Autodesk Inventor part; units mm, degrees
(part 3 of 5)
  line L1792 (36.1896, -14.5898) -> (36.2262, -14.8073)
  line L1793 (36.1751, -14.3579) -> (36.1896, -14.5898)
  line L1794 (36.1824, -14.1175) -> (36.1751, -14.3579)
  line L1795 (36.2227, -13.8474) -> (36.1824, -14.1175)
  line L1796 (36.3174, -13.5133) -> (36.2227, -13.8474)
  line L1797 (36.3367, -13.4614) -> (36.3174, -13.5133)
  line L1798 (36.3559, -13.4094) -> (36.3367, -13.4614)
  line L1799 (36.375, -13.3574) -> (36.3559, -13.4094)
  line L1800 (36.3941, -13.3053) -> (36.375, -13.3574)
  line L1801 (36.4131, -13.2533) -> (36.3941, -13.3053)
  circle A36 centre (0, 0) radius 4
  dimension "d26" = 8
  constraints: 3604 end point, 50 symmetric about line, 37 centre point, 4 midpoint, 1 coincident, 1 point on line, 1 other
  measures "d26" diameter of A36
extrude "押し出し1" add sketch "スケッチ1" along normal blind 3
sketch "スケッチ3" plane through (0, 0, 0) normal (0, 0, -1) x (-1, 0, 0)
  circle A0 centre (-26.7924, 20.9325) radius 1.6 projected
  circle A1 centre (-38.6125, 30.1674) radius 1.6 projected
  line L0 (-15.8708, 21.9173) -> (-25.1057, 10.0971) projected
  line L1 (-15.8708, 21.9173) -> (-140.3765, 119.1918) projected
  line L2 (-149.6114, 107.3716) -> (-140.3765, 119.1918) projected
  line L3 (-25.1057, 10.0971) -> (-149.6114, 107.3716) projected
  circle A2 centre (-9.3717, 32.6829) radius 1.6 projected
  circle A3 centre (-13.5062, 47.1018) radius 1.6 projected
  line L4 (0.0429, 27.0601) -> (-14.376, 22.9255) projected
  line L5 (0.0429, 27.0601) -> (-55.0846, 219.3124) projected
  line L6 (-69.5035, 215.1779) -> (-55.0846, 219.3124) projected
  line L7 (-14.376, 22.9255) -> (-69.5035, 215.1779) projected
  arc A4 (-9.1991, 59.2906) -> (-51.5273, 30.7399) centre (0, 0) ccw
  line L8 (-51.5273, 30.7399) -> (-25.1057, 10.0971)
  line L9 (-9.1991, 59.2906) -> (0.0429, 27.0601)
  line L10 (-25.1057, 10.0971) -> (0.0429, 27.0601)
  dimension "d23" = 60
  constraints: 6 end point, 2 point on circle, 2 point on line, 1 centre point, 1 coincident, 1 collinear, 1 perpendicular
  measures "d23" radius of A4
extrude "押し出し2" add sketch "スケッチ3" against normal blind 3 contours A0 | A1 | L1 A4 L7 L4 L10 L0 | L0 L3 A4 L1 | L4 L7 A4 L5 | A2 | A3
sketch "スケッチ2" plane through (0, 0, 0) normal (0, 0, -1) x (-1, 0, 0)
  line L0 (-25.1057, 10.0971) -> (-15.8708, 21.9173)
  line L1 (-15.8708, 21.9173) -> (-140.3765, 119.1918)
  line L2 (-140.3765, 119.1918) -> (-149.6114, 107.3716)
  line L3 (-149.6114, 107.3716) -> (-25.1057, 10.0971)
  line L4 (-20.4883, 16.0072) -> (0, 0)
  line L5 (0, 0) -> (0, 26)
  line L6 (0, 0) -> (-9.3717, 32.6829)
  point P0 (-26.7924, 20.9325)
  point P1 (-38.6125, 30.1674)
  point P2 (-13.5062, 47.1018)
  dimension "d6" = 158
  dimension "d7" = 15
  dimension "d8" = 52
  dimension "d9" = 26
  dimension "d10" = 15
  dimension "d11" = 8
  dimension "d42" = 15
  dimension "d43" = 34
  dimension "d44" = 36
  constraints: 14 end point, 3 point on line, 2 parallel, 2 perpendicular, 1 equal length, 1 midpoint, 1 vertical
  measures "d6" distance of L1.end L0.end
  measures "d7" distance of L1.end L2.end
  measures "d8" angle of L4 L5
  measures "d9" distance of L4.start L4.end
  measures "d10" distance of point (-38.613, 30.167) point (-26.792, 20.932)
  measures "d11" distance from line of point (-26.792, 20.932) L0
  measures "d42" distance of point (-13.506, 47.102) L6.end
  measures "d43" distance of L4.end L6.end
  measures "d44" angle of L4 L6
hole "穴1" at (26.7924, 20.9325, 0) at (38.6125, 30.1674, 0) at (9.3717, 32.6829, 0) at (13.5062, 47.1018, 0) direction (0, 0, 1) diameter 2.459 end through all thread size "M3x0.5" class "6H" standard "ISO Metric profile"
sketch "スケッチ4" plane through (0, 0, 0) normal (0, 0, -1) x (-1, 0, 0)
  circle A0 centre (-9.3717, 32.6829) radius 1.2295 projected
  circle A1 centre (-26.7924, 20.9325) radius 1.2295 projected
  circle A2 centre (-38.6125, 30.1674) radius 1.2295 projected
  circle A3 centre (-13.5062, 47.1018) radius 1.2295 projected
  line L0 (-43.4971, 24.2746) -> (-43.4223, 24.4075) projected
  line L1 (-43.6728, 23.957) -> (-43.4971, 24.2746) projected
  line L2 (-43.8463, 23.638) -> (-43.6728, 23.957) projected
  line L3 (-44.0174, 23.3178) -> (-43.8463, 23.638) projected
  line L4 (-43.7924, 22.9383) -> (-44.0174, 23.3178) projected
  line L5 (-43.5626, 22.5656) -> (-43.7924, 22.9383) projected
  line L6 (-43.3282, 22.1998) -> (-43.5626, 22.5656) projected
  line L7 (-43.0891, 21.841) -> (-43.3282, 22.1998) projected
  line L8 (-42.8453, 21.4895) -> (-43.0891, 21.841) projected
  line L9 (-42.5969, 21.1453) -> (-42.8453, 21.4895) projected
  line L10 (-42.3439, 20.8086) -> (-42.5969, 21.1453) projected
  line L11 (-42.0862, 20.4798) -> (-42.3439, 20.8086) projected
  line L12 (-41.8239, 20.1589) -> (-42.0862, 20.4798) projected
  line L13 (-41.5569, 19.8464) -> (-41.8239, 20.1589) projected
  line L14 (-41.2851, 19.5423) -> (-41.5569, 19.8464) projected
  line L15 (-41.0086, 19.2472) -> (-41.2851, 19.5423) projected
  line L16 (-40.7272, 18.9615) -> (-41.0086, 19.2472) projected
  line L17 (-40.4408, 18.6855) -> (-40.7272, 18.9615) projected
  line L18 (-40.1491, 18.4201) -> (-40.4408, 18.6855) projected
  line L19 (-39.852, 18.1659) -> (-40.1491, 18.4201) projected
  line L20 (-39.5489, 17.9241) -> (-39.852, 18.1659) projected
  line L21 (-39.2392, 17.6965) -> (-39.5489, 17.9241) projected
  line L22 (-38.9217, 17.4859) -> (-39.2392, 17.6965) projected
  line L23 (-38.5928, 17.3007) -> (-38.9217, 17.4859) projected
  line L24 (-38.3425, 17.1764) -> (-38.5928, 17.3007) projected
  line L25 (-38.105, 17.0451) -> (-38.3425, 17.1764) projected
  line L26 (-37.8794, 16.9086) -> (-38.105, 17.0451) projected
  line L27 (-37.6648, 16.7698) -> (-37.8794, 16.9086) projected
  line L28 (-37.4636, 16.6236) -> (-37.6648, 16.7698) projected
  line L29 (-37.2761, 16.4698) -> (-37.4636, 16.6236) projected
  line L30 (-37.1025, 16.3084) -> (-37.2761, 16.4698) projected
  line L31 (-36.9406, 16.1452) -> (-37.1025, 16.3084) projected
  line L32 (-36.7931, 15.9746) -> (-36.9406, 16.1452) projected
  line L33 (-36.6611, 15.7947) -> (-36.7931, 15.9746) projected
  line L34 (-36.5421, 15.6124) -> (-36.6611, 15.7947) projected
  line L35 (-36.4388, 15.4218) -> (-36.5421, 15.6124) projected
  line L36 (-36.3516, 15.2235) -> (-36.4388, 15.4218) projected
  line L37 (-36.2795, 15.0209) -> (-36.3516, 15.2235) projected
  line L38 (-36.2262, 14.8073) -> (-36.2795, 15.0209) projected
  line L39 (-36.1896, 14.5898) -> (-36.2262, 14.8073) projected
  line L40 (-36.1751, 14.3579) -> (-36.1896, 14.5898) projected
  line L41 (-36.1824, 14.1175) -> (-36.1751, 14.3579) projected
  line L42 (-36.2227, 13.8474) -> (-36.1824, 14.1175) projected
  line L43 (-36.3174, 13.5133) -> (-36.2227, 13.8474) projected
  line L44 (-36.3367, 13.4614) -> (-36.3174, 13.5133) projected
  line L45 (-36.3559, 13.4094) -> (-36.3367, 13.4614) projected
  line L46 (-36.375, 13.3574) -> (-36.3559, 13.4094) projected
  line L47 (-36.3941, 13.3053) -> (-36.375, 13.3574) projected
  line L48 (-36.4131, 13.2533) -> (-36.3941, 13.3053) projected
  line L49 (-36.432, 13.2012) -> (-36.4131, 13.2533) projected
  line L50 (-36.4508, 13.1491) -> (-36.432, 13.2012) projected
  line L51 (-36.4696, 13.0969) -> (-36.4508, 13.1491) projected
  line L52 (-36.4883, 13.0448) -> (-36.4696, 13.0969) projected
  line L53 (-36.5069, 12.9926) -> (-36.4883, 13.0448) projected
  line L54 (-36.6492, 12.6758) -> (-36.5069, 12.9926) projected
  line L55 (-36.7919, 12.4429) -> (-36.6492, 12.6758) projected
  line L56 (-36.9408, 12.2541) -> (-36.7919, 12.4429) projected
  line L57 (-37.1009, 12.0858) -> (-36.9408, 12.2541) projected
  line L58 (-37.2688, 11.9427) -> (-37.1009, 12.0858) projected
  line L59 (-37.447, 11.8133) -> (-37.2688, 11.9427) projected
  line L60 (-37.6324, 11.7044) -> (-37.447, 11.8133) projected
  line L61 (-37.8267, 11.6087) -> (-37.6324, 11.7044) projected
  line L62 (-38.0283, 11.529) -> (-37.8267, 11.6087) projected
  line L63 (-38.2367, 11.4659) -> (-38.0283, 11.529) projected
  line L64 (-38.4534, 11.4129) -> (-38.2367, 11.4659) projected
  line L65 (-38.6761, 11.377) -> (-38.4534, 11.4129) projected
  line L66 (-38.905, 11.3561) -> (-38.6761, 11.377) projected
  line L67 (-39.1417, 11.344) -> (-38.905, 11.3561) projected
  line L68 (-39.3842, 11.3467) -> (-39.1417, 11.344) projected
  line L69 (-39.6323, 11.364) -> (-39.3842, 11.3467) projected
  line L70 (-39.886, 11.3956) -> (-39.6323, 11.364) projected
  line L71 (-40.1465, 11.4361) -> (-39.886, 11.3956) projected
  line L72 (-40.4129, 11.4882) -> (-40.1465, 11.4361) projected
  line L73 (-40.6845, 11.5538) -> (-40.4129, 11.4882) projected
  line L74 (-41.0555, 11.6234) -> (-40.6845, 11.5538) projected
  line L75 (-41.4341, 11.6662) -> (-41.0555, 11.6234) projected
  line L76 (-41.8176, 11.6908) -> (-41.4341, 11.6662) projected
  line L77 (-42.2052, 11.7005) -> (-41.8176, 11.6908) projected
  line L78 (-42.5962, 11.6968) -> (-42.2052, 11.7005) projected
  line L79 (-42.9903, 11.6809) -> (-42.5962, 11.6968) projected
  line L80 (-43.387, 11.6536) -> (-42.9903, 11.6809) projected
  line L81 (-43.7863, 11.6156) -> (-43.387, 11.6536) projected
  line L82 (-44.1878, 11.5673) -> (-43.7863, 11.6156) projected
  line L83 (-44.5914, 11.509) -> (-44.1878, 11.5673) projected
  line L84 (-44.9969, 11.4412) -> (-44.5914, 11.509) projected
  line L85 (-45.4041, 11.3641) -> (-44.9969, 11.4412) projected
  line L86 (-45.8128, 11.2778) -> (-45.4041, 11.3641) projected
  line L87 (-46.223, 11.1825) -> (-45.8128, 11.2778) projected
  line L88 (-46.6346, 11.0786) -> (-46.223, 11.1825) projected
  line L89 (-47.0473, 10.9659) -> (-46.6346, 11.0786) projected
  line L90 (-47.4611, 10.8448) -> (-47.0473, 10.9659) projected
  line L91 (-47.8758, 10.7152) -> (-47.4611, 10.8448) projected
  line L92 (-48.2914, 10.5774) -> (-47.8758, 10.7152) projected
  line L93 (-48.7077, 10.4313) -> (-48.2914, 10.5774) projected
  line L94 (-48.7824, 10.0761) -> (-48.7077, 10.4313) projected
  line L95 (-48.8546, 9.7203) -> (-48.7824, 10.0761) projected
  line L96 (-48.9241, 9.3639) -> (-48.8546, 9.7203) projected
  line L97 (-48.9911, 9.0071) -> (-48.9241, 9.3639) projected
  line L98 (-49.0554, 8.6498) -> (-48.9911, 9.0071) projected
  line L99 (-49.1172, 8.292) -> (-49.0554, 8.6498) projected
  line L100 (-49.1763, 7.9338) -> (-49.1172, 8.292) projected
  line L101 (-49.2328, 7.5752) -> (-49.1763, 7.9338) projected
  line L102 (-49.2867, 7.2162) -> (-49.2328, 7.5752) projected
  line L103 (-49.338, 6.8568) -> (-49.2867, 7.2162) projected
  line L104 (-48.9968, 6.5771) -> (-49.338, 6.8568) projected
  line L105 (-48.6534, 6.3055) -> (-48.9968, 6.5771) projected
  line L106 (-48.308, 6.0419) -> (-48.6534, 6.3055) projected
  line L107 (-47.9606, 5.7865) -> (-48.308, 6.0419) projected
  line L108 (-47.6113, 5.5395) -> (-47.9606, 5.7865) projected
  line L109 (-47.2601, 5.3011) -> (-47.6113, 5.5395) projected
  line L110 (-46.9072, 5.0713) -> (-47.2601, 5.3011) projected
  line L111 (-46.5526, 4.8504) -> (-46.9072, 5.0713) projected
  line L112 (-46.1963, 4.6386) -> (-46.5526, 4.8504) projected
  line L113 (-45.8385, 4.4362) -> (-46.1963, 4.6386) projected
  line L114 (-45.4792, 4.2434) -> (-45.8385, 4.4362) projected
  line L115 (-45.1184, 4.0607) -> (-45.4792, 4.2434) projected
  line L116 (-44.7563, 3.8884) -> (-45.1184, 4.0607) projected
  line L117 (-44.3927, 3.7271) -> (-44.7563, 3.8884) projected
  line L118 (-44.0279, 3.5774) -> (-44.3927, 3.7271) projected
  line L119 (-43.6617, 3.4402) -> (-44.0279, 3.5774) projected
  line L120 (-43.2942, 3.3167) -> (-43.6617, 3.4402) projected
  line L121 (-42.9254, 3.2087) -> (-43.2942, 3.3167) projected
  line L122 (-42.555, 3.1194) -> (-42.9254, 3.2087) projected
  line L123 (-42.1825, 3.0578) -> (-42.555, 3.1194) projected
  line L124 (-41.9049, 3.0266) -> (-42.1825, 3.0578) projected
  line L125 (-41.6367, 2.9845) -> (-41.9049, 3.0266) projected
  line L126 (-41.3781, 2.9334) -> (-41.6367, 2.9845) projected
  line L127 (-41.1289, 2.8764) -> (-41.3781, 2.9334) projected
  line L128 (-40.8898, 2.8078) -> (-41.1289, 2.8764) projected
  line L129 (-40.661, 2.7274) -> (-40.8898, 2.8078) projected
  line L130 (-40.4428, 2.6351) -> (-40.661, 2.7274) projected
  line L131 (-40.2348, 2.5371) -> (-40.4428, 2.6351) projected
  line L132 (-40.0379, 2.4272) -> (-40.2348, 2.5371) projected
  line L133 (-39.8523, 2.3033) -> (-40.0379, 2.4272) projected
  line L134 (-39.6781, 2.1727) -> (-39.8523, 2.3033) projected
  line L135 (-39.5158, 2.0289) -> (-39.6781, 2.1727) projected
  line L136 (-39.366, 1.8725) -> (-39.5158, 2.0289) projected
  line L137 (-39.2291, 1.7067) -> (-39.366, 1.8725) projected
  line L138 (-39.1059, 1.5242) -> (-39.2291, 1.7067) projected
  line L139 (-38.997, 1.3323) -> (-39.1059, 1.5242) projected
  line L140 (-38.9042, 1.1194) -> (-38.997, 1.3323) projected
  line L141 (-38.8288, 0.891) -> (-38.9042, 1.1194) projected
  line L142 (-38.7743, 0.6234) -> (-38.8288, 0.891) projected
  line L143 (-38.749, 0.2771) -> (-38.7743, 0.6234) projected
  line L144 (-38.7494, 0.2217) -> (-38.749, 0.2771) projected
  line L145 (-38.7496, 0.1663) -> (-38.7494, 0.2217) projected
  line L146 (-38.7498, 0.1108) -> (-38.7496, 0.1663) projected
  line L147 (-38.75, 0.0554) -> (-38.7498, 0.1108) projected
  line L148 (-38.75, 0) -> (-38.75, 0.0554) projected
  line L149 (-38.75, -0.0554) -> (-38.75, 0) projected
  line L150 (-38.7498, -0.1108) -> (-38.75, -0.0554) projected
  line L151 (-38.7496, -0.1663) -> (-38.7498, -0.1108) projected
  line L152 (-38.7494, -0.2217) -> (-38.7496, -0.1663) projected
  line L153 (-38.749, -0.2771) -> (-38.7494, -0.2217) projected
  line L154 (-38.7743, -0.6234) -> (-38.749, -0.2771) projected
  line L155 (-38.8288, -0.891) -> (-38.7743, -0.6234) projected
  line L156 (-38.9042, -1.1194) -> (-38.8288, -0.891) projected
  line L157 (-38.997, -1.3323) -> (-38.9042, -1.1194) projected
  line L158 (-39.1059, -1.5242) -> (-38.997, -1.3323) projected
  line L159 (-39.2291, -1.7067) -> (-39.1059, -1.5242) projected
  line L160 (-39.366, -1.8725) -> (-39.2291, -1.7067) projected
  line L161 (-39.5158, -2.0289) -> (-39.366, -1.8725) projected
  line L162 (-39.6781, -2.1727) -> (-39.5158, -2.0289) projected
  line L163 (-39.8523, -2.3033) -> (-39.6781, -2.1727) projected
  line L164 (-40.0379, -2.4272) -> (-39.8523, -2.3033) projected
  line L165 (-40.2348, -2.5371) -> (-40.0379, -2.4272) projected
  line L166 (-40.4428, -2.6351) -> (-40.2348, -2.5371) projected
  line L167 (-40.661, -2.7274) -> (-40.4428, -2.6351) projected
  line L168 (-40.8898, -2.8078) -> (-40.661, -2.7274) projected
  line L169 (-41.1289, -2.8764) -> (-40.8898, -2.8078) projected
  line L170 (-41.3781, -2.9334) -> (-41.1289, -2.8764) projected
  line L171 (-41.6367, -2.9845) -> (-41.3781, -2.9334) projected
  line L172 (-41.9049, -3.0266) -> (-41.6367, -2.9845) projected
  line L173 (-42.1825, -3.0578) -> (-41.9049, -3.0266) projected
  line L174 (-42.555, -3.1194) -> (-42.1825, -3.0578) projected
  line L175 (-42.9254, -3.2087) -> (-42.555, -3.1194) projected
  line L176 (-43.2942, -3.3167) -> (-42.9254, -3.2087) projected
  line L177 (-43.6617, -3.4402) -> (-43.2942, -3.3167) projected
  line L178 (-44.0279, -3.5774) -> (-43.6617, -3.4402) projected
  line L179 (-44.3927, -3.7271) -> (-44.0279, -3.5774) projected
  line L180 (-44.7563, -3.8884) -> (-44.3927, -3.7271) projected
  line L181 (-45.1184, -4.0607) -> (-44.7563, -3.8884) projected
  line L182 (-45.4792, -4.2434) -> (-45.1184, -4.0607) projected
  line L183 (-45.8385, -4.4362) -> (-45.4792, -4.2434) projected
  line L184 (-46.1963, -4.6386) -> (-45.8385, -4.4362) projected
  line L185 (-46.5526, -4.8504) -> (-46.1963, -4.6386) projected
  line L186 (-46.9072, -5.0713) -> (-46.5526, -4.8504) projected
  line L187 (-47.2601, -5.3011) -> (-46.9072, -5.0713) projected
  line L188 (-47.6113, -5.5395) -> (-47.2601, -5.3011) projected
  line L189 (-47.9606, -5.7865) -> (-47.6113, -5.5395) projected
  line L190 (-48.308, -6.0419) -> (-47.9606, -5.7865) projected
  line L191 (-48.6534, -6.3055) -> (-48.308, -6.0419) projected
  line L192 (-48.9968, -6.5771) -> (-48.6534, -6.3055) projected
  line L193 (-49.338, -6.8568) -> (-48.9968, -6.5771) projected
  line L194 (-49.2867, -7.2162) -> (-49.338, -6.8568) projected
  line L195 (-49.2328, -7.5752) -> (-49.2867, -7.2162) projected
  line L196 (-49.1763, -7.9338) -> (-49.2328, -7.5752) projected
  line L197 (-49.1172, -8.292) -> (-49.1763, -7.9338) projected
  line L198 (-49.0554, -8.6498) -> (-49.1172, -8.292) projected
  line L199 (-48.9911, -9.0071) -> (-49.0554, -8.6498) projected
  line L200 (-48.9241, -9.3639) -> (-48.9911, -9.0071) projected
  line L201 (-48.8546, -9.7203) -> (-48.9241, -9.3639) projected
  line L202 (-48.7824, -10.0761) -> (-48.8546, -9.7203) projected
  line L203 (-48.7077, -10.4313) -> (-48.7824, -10.0761) projected
  line L204 (-48.2914, -10.5774) -> (-48.7077, -10.4313) projected
  line L205 (-47.8758, -10.7152) -> (-48.2914, -10.5774) projected
  line L206 (-47.4611, -10.8448) -> (-47.8758, -10.7152) projected
  line L207 (-47.0473, -10.9659) -> (-47.4611, -10.8448) projected
  line L208 (-46.6346, -11.0786) -> (-47.0473, -10.9659) projected
  line L209 (-46.223, -11.1825) -> (-46.6346, -11.0786) projected
  line L210 (-45.8128, -11.2778) -> (-46.223, -11.1825) projected
  line L211 (-45.4041, -11.3641) -> (-45.8128, -11.2778) projected
  line L212 (-44.9969, -11.4412) -> (-45.4041, -11.3641) projected
  line L213 (-44.5914, -11.509) -> (-44.9969, -11.4412) projected
  line L214 (-44.1878, -11.5673) -> (-44.5914, -11.509) projected
  line L215 (-43.7863, -11.6156) -> (-44.1878, -11.5673) projected
  line L216 (-43.387, -11.6536) -> (-43.7863, -11.6156) projected
  line L217 (-42.9903, -11.6809) -> (-43.387, -11.6536) projected
  line L218 (-42.5962, -11.6968) -> (-42.9903, -11.6809) projected
  line L219 (-42.2052, -11.7005) -> (-42.5962, -11.6968) projected
  line L220 (-41.8176, -11.6908) -> (-42.2052, -11.7005) projected
  line L221 (-41.4341, -11.6662) -> (-41.8176, -11.6908) projected
  line L222 (-41.0555, -11.6234) -> (-41.4341, -11.6662) projected
  line L223 (-40.6845, -11.5538) -> (-41.0555, -11.6234) projected
  line L224 (-40.4129, -11.4882) -> (-40.6845, -11.5538) projected
  line L225 (-40.1465, -11.4361) -> (-40.4129, -11.4882) projected
  line L226 (-39.886, -11.3956) -> (-40.1465, -11.4361) projected
  line L227 (-39.6323, -11.364) -> (-39.886, -11.3956) projected
  line L228 (-39.3842, -11.3467) -> (-39.6323, -11.364) projected
  line L229 (-39.1417, -11.344) -> (-39.3842, -11.3467) projected
  line L230 (-38.905, -11.3561) -> (-39.1417, -11.344) projected
  line L231 (-38.6761, -11.377) -> (-38.905, -11.3561) projected
  line L232 (-38.4534, -11.4129) -> (-38.6761, -11.377) projected
  line L233 (-38.2367, -11.4659) -> (-38.4534, -11.4129) projected
  line L234 (-38.0283, -11.529) -> (-38.2367, -11.4659) projected
  line L235 (-37.8267, -11.6087) -> (-38.0283, -11.529) projected
  line L236 (-37.6324, -11.7044) -> (-37.8267, -11.6087) projected
  line L237 (-37.447, -11.8133) -> (-37.6324, -11.7044) projected
  line L238 (-37.2688, -11.9427) -> (-37.447, -11.8133) projected
  line L239 (-37.1009, -12.0858) -> (-37.2688, -11.9427) projected
  line L240 (-36.9408, -12.2541) -> (-37.1009, -12.0858) projected
  line L241 (-36.7919, -12.4429) -> (-36.9408, -12.2541) projected
  line L242 (-36.6492, -12.6758) -> (-36.7919, -12.4429) projected
  line L243 (-36.5069, -12.9926) -> (-36.6492, -12.6758) projected
  line L244 (-36.4883, -13.0448) -> (-36.5069, -12.9926) projected
  line L245 (-36.4696, -13.0969) -> (-36.4883, -13.0448) projected
  line L246 (-36.4508, -13.1491) -> (-36.4696, -13.0969) projected
  line L247 (-36.432, -13.2012) -> (-36.4508, -13.1491) projected
  line L248 (-36.4131, -13.2533) -> (-36.432, -13.2012) projected
  line L249 (-36.3941, -13.3053) -> (-36.4131, -13.2533) projected
  line L250 (-36.375, -13.3574) -> (-36.3941, -13.3053) projected
  line L251 (-36.3559, -13.4094) -> (-36.375, -13.3574) projected
  line L252 (-36.3367, -13.4614) -> (-36.3559, -13.4094) projected
  line L253 (-36.3174, -13.5133) -> (-36.3367, -13.4614) projected
  line L254 (-36.2227, -13.8474) -> (-36.3174, -13.5133) projected
  line L255 (-36.1824, -14.1175) -> (-36.2227, -13.8474) projected
  line L256 (-36.1751, -14.3579) -> (-36.1824, -14.1175) projected
  line L257 (-36.1896, -14.5898) -> (-36.1751, -14.3579) projected
  line L258 (-36.2262, -14.8073) -> (-36.1896, -14.5898) projected
  line L259 (-36.2795, -15.0209) -> (-36.2262, -14.8073) projected
  line L260 (-36.3516, -15.2235) -> (-36.2795, -15.0209) projected
  line L261 (-36.4388, -15.4218) -> (-36.3516, -15.2235) projected
  line L262 (-36.5421, -15.6124) -> (-36.4388, -15.4218) projected
  line L263 (-36.6611, -15.7947) -> (-36.5421, -15.6124) projected
  line L264 (-36.7931, -15.9746) -> (-36.6611, -15.7947) projected
  line L265 (-36.9406, -16.1452) -> (-36.7931, -15.9746) projected
  line L266 (-37.1025, -16.3084) -> (-36.9406, -16.1452) projected
  line L267 (-37.2761, -16.4698) -> (-37.1025, -16.3084) projected
  line L268 (-37.4636, -16.6236) -> (-37.2761, -16.4698) projected
  line L269 (-37.6648, -16.7698) -> (-37.4636, -16.6236) projected
  line L270 (-37.8794, -16.9086) -> (-37.6648, -16.7698) projected
  line L271 (-38.105, -17.0451) -> (-37.8794, -16.9086) projected
  line L272 (-38.3425, -17.1764) -> (-38.105, -17.0451) projected
  line L273 (-38.5928, -17.3007) -> (-38.3425, -17.1764) projected
  line L274 (-38.9217, -17.4859) -> (-38.5928, -17.3007) projected
  line L275 (-39.2392, -17.6965) -> (-38.9217, -17.4859) projected
  line L276 (-39.5489, -17.9241) -> (-39.2392, -17.6965) projected
  line L277 (-39.852, -18.1659) -> (-39.5489, -17.9241) projected
  line L278 (-40.1491, -18.4201) -> (-39.852, -18.1659) projected
  line L279 (-40.4408, -18.6855) -> (-40.1491, -18.4201) projected
  line L280 (-40.7272, -18.9615) -> (-40.4408, -18.6855) projected
  line L281 (-41.0086, -19.2472) -> (-40.7272, -18.9615) projected
  line L282 (-41.2851, -19.5423) -> (-41.0086, -19.2472) projected
  line L283 (-41.5569, -19.8464) -> (-41.2851, -19.5423) projected
  line L284 (-41.8239, -20.1589) -> (-41.5569, -19.8464) projected
  line L285 (-42.0862, -20.4798) -> (-41.8239, -20.1589) projected
  line L286 (-42.3439, -20.8086) -> (-42.0862, -20.4798) projected
  line L287 (-42.5969, -21.1453) -> (-42.3439, -20.8086) projected
  line L288 (-42.8453, -21.4895) -> (-42.5969, -21.1453) projected
  line L289 (-43.0891, -21.841) -> (-42.8453, -21.4895) projected
  line L290 (-43.3282, -22.1998) -> (-43.0891, -21.841) projected
  line L291 (-43.5626, -22.5656) -> (-43.3282, -22.1998) projected
  line L292 (-43.7924, -22.9383) -> (-43.5626, -22.5656) projected
  line L293 (-44.0174, -23.3178) -> (-43.7924, -22.9383) projected
  line L294 (-43.8463, -23.638) -> (-44.0174, -23.3178) projected
  line L295 (-43.6728, -23.957) -> (-43.8463, -23.638) projected
  line L296 (-43.4971, -24.2746) -> (-43.6728, -23.957) projected
  line L297 (-43.319, -24.591) -> (-43.4971, -24.2746) projected
  line L298 (-43.1386, -24.9061) -> (-43.319, -24.591) projected
  line L299 (-42.9559, -25.2198) -> (-43.1386, -24.9061) projected
  line L300 (-42.771, -25.5322) -> (-42.9559, -25.2198) projected
  line L301 (-42.5838, -25.8433) -> (-42.771, -25.5322) projected
  line L302 (-42.3943, -26.153) -> (-42.5838, -25.8433) projected
  line L303 (-42.2025, -26.4613) -> (-42.3943, -26.153) projected
  line L304 (-41.7614, -26.4561) -> (-42.2025, -26.4613) projected
  line L305 (-41.3237, -26.4435) -> (-41.7614, -26.4561) projected
  line L306 (-40.8897, -26.4234) -> (-41.3237, -26.4435) projected
  line L307 (-40.4594, -26.3957) -> (-40.8897, -26.4234) projected
  line L308 (-40.0331, -26.3604) -> (-40.4594, -26.3957) projected
  line L309 (-39.6108, -26.3174) -> (-40.0331, -26.3604) projected
  line L310 (-39.1928, -26.2665) -> (-39.6108, -26.3174) projected
  line L311 (-38.7791, -26.2078) -> (-39.1928, -26.2665) projected
  line L312 (-38.3701, -26.1411) -> (-38.7791, -26.2078) projected
  line L313 (-37.9659, -26.0661) -> (-38.3701, -26.1411) projected
  line L314 (-37.5667, -25.9828) -> (-37.9659, -26.0661) projected
  line L315 (-37.1729, -25.8909) -> (-37.5667, -25.9828) projected
  line L316 (-36.7847, -25.7901) -> (-37.1729, -25.8909) projected
  line L317 (-36.4025, -25.68) -> (-36.7847, -25.7901) projected
  line L318 (-36.0268, -25.5601) -> (-36.4025, -25.68) projected
  line L319 (-35.6581, -25.4299) -> (-36.0268, -25.5601) projected
  line L320 (-35.2972, -25.2883) -> (-35.6581, -25.4299) projected
  line L321 (-34.9452, -25.1339) -> (-35.2972, -25.2883) projected
  line L322 (-34.6041, -24.9642) -> (-34.9452, -25.1339) projected
  line L323 (-34.2792, -24.772) -> (-34.6041, -24.9642) projected
  line L324 (-34.0465, -24.6174) -> (-34.2792, -24.772) projected
  line L325 (-33.814, -24.4773) -> (-34.0465, -24.6174) projected
  line L326 (-33.583, -24.3502) -> (-33.814, -24.4773) projected
  line L327 (-33.3555, -24.2337) -> (-33.583, -24.3502) projected
  line L328 (-33.1282, -24.1326) -> (-33.3555, -24.2337) projected
  line L329 (-32.9013, -24.0471) -> (-33.1282, -24.1326) projected
  line L330 (-32.6748, -23.9775) -> (-32.9013, -24.0471) projected
  line L331 (-32.4525, -23.9189) -> (-32.6748, -23.9775) projected
  line L332 (-32.231, -23.8765) -> (-32.4525, -23.9189) projected
  line L333 (-32.0092, -23.8521) -> (-32.231, -23.8765) projected
  line L334 (-31.7918, -23.8401) -> (-32.0092, -23.8521) projected
  line L335 (-31.575, -23.8461) -> (-31.7918, -23.8401) projected
  line L336 (-31.3597, -23.8696) -> (-31.575, -23.8461) projected
  line L337 (-31.1483, -23.9085) -> (-31.3597, -23.8696) projected
  line L338 (-30.9366, -23.9692) -> (-31.1483, -23.9085) projected
  line L339 (-30.7299, -24.0462) -> (-30.9366, -23.9692) projected
  line L340 (-30.5219, -24.1496) -> (-30.7299, -24.0462) projected
  line L341 (-30.3173, -24.2761) -> (-30.5219, -24.1496) projected
  line L342 (-30.1036, -24.4461) -> (-30.3173, -24.2761) projected
  line L343 (-29.8616, -24.6951) -> (-30.1036, -24.4461) projected
  line L344 (-29.8262, -24.7378) -> (-29.8616, -24.6951) projected
  line L345 (-29.7908, -24.7804) -> (-29.8262, -24.7378) projected
  line L346 (-29.7553, -24.823) -> (-29.7908, -24.7804) projected
  line L347 (-29.7198, -24.8655) -> (-29.7553, -24.823) projected
  line L348 (-29.6842, -24.908) -> (-29.7198, -24.8655) projected
  line L349 (-29.6486, -24.9504) -> (-29.6842, -24.908) projected
  line L350 (-29.6129, -24.9928) -> (-29.6486, -24.9504) projected
  line L351 (-29.5771, -25.0351) -> (-29.6129, -24.9928) projected
  line L352 (-29.5412, -25.0774) -> (-29.5771, -25.0351) projected
  line L353 (-29.5054, -25.1196) -> (-29.5412, -25.0774) projected
  line L354 (-29.3021, -25.4012) -> (-29.5054, -25.1196) projected
  line L355 (-29.1718, -25.6412) -> (-29.3021, -25.4012) projected
  line L356 (-29.0828, -25.8646) -> (-29.1718, -25.6412) projected
  line L357 (-29.0171, -26.0875) -> (-29.0828, -25.8646) projected
  line L358 (-28.9771, -26.3044) -> (-29.0171, -26.0875) projected
  line L359 (-28.9541, -26.5234) -> (-28.9771, -26.3044) projected
  line L360 (-28.9525, -26.7384) -> (-28.9541, -26.5234) projected
  line L361 (-28.9667, -26.9545) -> (-28.9525, -26.7384) projected
  line L362 (-28.9985, -27.169) -> (-28.9667, -26.9545) projected
  line L363 (-29.0481, -27.381) -> (-28.9985, -27.169) projected
  line L364 (-29.1106, -27.5952) -> (-29.0481, -27.381) projected
  line L365 (-29.1908, -27.806) -> (-29.1106, -27.5952) projected
  line L366 (-29.2872, -28.0147) -> (-29.1908, -27.806) projected
  line L367 (-29.395, -28.2257) -> (-29.2872, -28.0147) projected
  line L368 (-29.5186, -28.4343) -> (-29.395, -28.2257) projected
  line L369 (-29.6577, -28.6406) -> (-29.5186, -28.4343) projected
  line L370 (-29.8119, -28.8444) -> (-29.6577, -28.6406) projected
  line L371 (-29.9772, -29.0498) -> (-29.8119, -28.8444) projected
  line L372 (-30.1555, -29.2545) -> (-29.9772, -29.0498) projected
  line L373 (-30.3482, -29.4569) -> (-30.1555, -29.2545) projected
  line L374 (-30.5939, -29.7434) -> (-30.3482, -29.4569) projected
  line L375 (-30.8202, -30.0499) -> (-30.5939, -29.7434) projected
  line L376 (-31.0334, -30.3697) -> (-30.8202, -30.0499) projected
  line L377 (-31.2355, -30.7005) -> (-31.0334, -30.3697) projected
  line L378 (-31.4278, -31.041) -> (-31.2355, -30.7005) projected
  line L379 (-31.6111, -31.3902) -> (-31.4278, -31.041) projected
  line L380 (-31.7858, -31.7475) -> (-31.6111, -31.3902) projected
  line L381 (-31.9525, -32.1123) -> (-31.7858, -31.7475) projected
  line L382 (-32.1115, -32.4841) -> (-31.9525, -32.1123) projected
  line L383 (-32.2628, -32.8628) -> (-32.1115, -32.4841) projected
  line L384 (-32.4068, -33.2478) -> (-32.2628, -32.8628) projected
  line L385 (-32.5436, -33.639) -> (-32.4068, -33.2478) projected
  line L386 (-32.6732, -34.0362) -> (-32.5436, -33.639) projected
  line L387 (-32.7959, -34.4391) -> (-32.6732, -34.0362) projected
  line L388 (-32.9116, -34.8475) -> (-32.7959, -34.4391) projected
  line L389 (-33.0204, -35.2612) -> (-32.9116, -34.8475) projected
  line L390 (-33.1224, -35.6801) -> (-33.0204, -35.2612) projected
  line L391 (-33.2176, -36.1041) -> (-33.1224, -35.6801) projected
  line L392 (-33.306, -36.5329) -> (-33.2176, -36.1041) projected
  line L393 (-33.3877, -36.9664) -> (-33.306, -36.5329) projected
  line L394 (-33.1173, -37.2088) -> (-33.3877, -36.9664) projected
  line L395 (-32.8453, -37.4492) -> (-33.1173, -37.2088) projected
  line L396 (-32.5715, -37.6876) -> (-32.8453, -37.4492) projected
  line L397 (-32.2959, -37.924) -> (-32.5715, -37.6876) projected
  line L398 (-32.0186, -38.1583) -> (-32.2959, -37.924) projected
  line L399 (-31.7397, -38.3907) -> (-32.0186, -38.1583) projected
  line L400 (-31.459, -38.621) -> (-31.7397, -38.3907) projected
  line L401 (-31.1767, -38.8493) -> (-31.459, -38.621) projected
  line L402 (-30.8927, -39.0755) -> (-31.1767, -38.8493) projected
  line L403 (-30.6071, -39.2996) -> (-30.8927, -39.0755) projected
  line L404 (-30.1943, -39.1439) -> (-30.6071, -39.2996) projected
  line L405 (-29.7874, -38.9823) -> (-30.1943, -39.1439) projected
  line L406 (-29.3864, -38.815) -> (-29.7874, -38.9823) projected
  line L407 (-28.9916, -38.6418) -> (-29.3864, -38.815) projected
  line L408 (-28.603, -38.4628) -> (-28.9916, -38.6418) projected
  line L409 (-28.2209, -38.2779) -> (-28.603, -38.4628) projected
  line L410 (-27.8455, -38.0872) -> (-28.2209, -38.2779) projected
  line L411 (-27.4768, -37.8905) -> (-27.8455, -38.0872) projected
  line L412 (-27.1153, -37.6879) -> (-27.4768, -37.8905) projected
  line L413 (-26.7611, -37.4792) -> (-27.1153, -37.6879) projected
  line L414 (-26.4145, -37.2644) -> (-26.7611, -37.4792) projected
  line L415 (-26.0759, -37.0434) -> (-26.4145, -37.2644) projected
  line L416 (-25.7456, -36.8158) -> (-26.0759, -37.0434) projected
  line L417 (-25.4241, -36.5817) -> (-25.7456, -36.8158) projected
  line L418 (-25.1121, -36.3405) -> (-25.4241, -36.5817) projected
  line L419 (-24.8101, -36.092) -> (-25.1121, -36.3405) projected
  line L420 (-24.5194, -35.8356) -> (-24.8101, -36.092) projected
  line L421 (-24.2415, -35.5701) -> (-24.5194, -35.8356) projected
  line L422 (-23.979, -35.294) -> (-24.2415, -35.5701) projected
  line L423 (-23.7394, -35.0022) -> (-23.979, -35.294) projected
  line L424 (-23.5736, -34.7774) -> (-23.7394, -35.0022) projected
  line L425 (-23.403, -34.5662) -> (-23.5736, -34.7774) projected
  line L426 (-23.2294, -34.3678) -> (-23.403, -34.5662) projected
  line L427 (-23.0555, -34.1805) -> (-23.2294, -34.3678) projected
  line L428 (-22.8765, -34.0078) -> (-23.0555, -34.1805) projected
  line L429 (-22.6925, -33.8498) -> (-22.8765, -34.0078) projected
  line L430 (-22.5034, -33.7069) -> (-22.6925, -33.8498) projected
  line L431 (-22.3146, -33.5758) -> (-22.5034, -33.7069) projected
  line L432 (-22.121, -33.4602) -> (-22.3146, -33.5758) projected
  line L433 (-21.9209, -33.3615) -> (-22.121, -33.4602) projected
  line L434 (-21.7207, -33.2758) -> (-21.9209, -33.3615) projected
  line L435 (-21.515, -33.2073) -> (-21.7207, -33.2758) projected
  line L436 (-21.3046, -33.1558) -> (-21.515, -33.2073) projected
  line L437 (-21.0926, -33.12) -> (-21.3046, -33.1558) projected
  line L438 (-20.8729, -33.1046) -> (-21.0926, -33.12) projected
  line L439 (-20.6524, -33.1063) -> (-20.8729, -33.1046) projected
  line L440 (-20.4215, -33.1323) -> (-20.6524, -33.1063) projected
  line L441 (-20.186, -33.1812) -> (-20.4215, -33.1323) projected
  line L442 (-19.9271, -33.2679) -> (-20.186, -33.1812) projected
  line L443 (-19.6145, -33.4191) -> (-19.9271, -33.2679) projected
  line L444 (-19.5667, -33.4471) -> (-19.6145, -33.4191) projected
  line L445 (-19.5188, -33.475) -> (-19.5667, -33.4471) projected
  line L446 (-19.4709, -33.5029) -> (-19.5188, -33.475) projected
  line L447 (-19.423, -33.5307) -> (-19.4709, -33.5029) projected
  line L448 (-19.375, -33.5585) -> (-19.423, -33.5307) projected
  line L449 (-19.327, -33.5862) -> (-19.375, -33.5585) projected
  line L450 (-19.2789, -33.6138) -> (-19.327, -33.5862) projected
  line L451 (-19.2308, -33.6413) -> (-19.2789, -33.6138) projected
  line L452 (-19.1827, -33.6688) -> (-19.2308, -33.6413) projected
  line L453 (-19.1345, -33.6962) -> (-19.1827, -33.6688) projected
  line L454 (-18.8473, -33.8913) -> (-19.1345, -33.6962) projected
  line L455 (-18.6427, -34.0722) -> (-18.8473, -33.8913) projected
  line L456 (-18.4826, -34.2517) -> (-18.6427, -34.0722) projected
  line L457 (-18.3447, -34.4386) -> (-18.4826, -34.2517) projected
  line L458 (-18.2329, -34.6288) -> (-18.3447, -34.4386) projected
  line L459 (-18.1365, -34.8267) -> (-18.2329, -34.6288) projected
  line L460 (-18.0614, -35.0282) -> (-18.1365, -34.8267) projected
  line L461 (-18.0008, -35.2362) -> (-18.0614, -35.0282) projected
  line L462 (-17.9574, -35.4486) -> (-18.0008, -35.2362) projected
  line L463 (-17.9314, -35.6648) -> (-17.9574, -35.4486) projected
  line L464 (-17.9169, -35.8874) -> (-17.9314, -35.6648) projected
  line L465 (-17.9202, -36.1129) -> (-17.9169, -35.8874) projected
  line L466 (-17.9393, -36.342) -> (-17.9202, -36.1129) projected
  line L467 (-17.9685, -36.5772) -> (-17.9393, -36.342) projected
  line L468 (-18.0133, -36.8155) -> (-17.9685, -36.5772) projected
  line L469 (-18.0734, -37.0569) -> (-18.0133, -36.8155) projected
  line L470 (-18.1486, -37.3012) -> (-18.0734, -37.0569) projected
  line L471 (-18.2337, -37.5507) -> (-18.1486, -37.3012) projected
  line L472 (-18.3313, -37.804) -> (-18.2337, -37.5507) projected
  line L473 (-18.4431, -38.0601) -> (-18.3313, -37.804) projected
  line L474 (-18.576, -38.4134) -> (-18.4431, -38.0601) projected
  line L475 (-18.6839, -38.7788) -> (-18.576, -38.4134) projected
  line L476 (-18.7748, -39.1522) -> (-18.6839, -38.7788) projected
  line L477 (-18.8516, -39.5322) -> (-18.7748, -39.1522) projected
  line L478 (-18.9158, -39.9179) -> (-18.8516, -39.5322) projected
  line L479 (-18.9686, -40.3088) -> (-18.9158, -39.9179) projected
  line L480 (-19.0107, -40.7043) -> (-18.9686, -40.3088) projected
  line L481 (-19.0425, -41.1041) -> (-19.0107, -40.7043) projected
  line L482 (-19.0647, -41.5079) -> (-19.0425, -41.1041) projected
  line L483 (-19.0774, -41.9154) -> (-19.0647, -41.5079) projected
  line L484 (-19.081, -42.3265) -> (-19.0774, -41.9154) projected
  line L485 (-19.0757, -42.7409) -> (-19.081, -42.3265) projected
  line L486 (-19.0617, -43.1585) -> (-19.0757, -42.7409) projected
  line L487 (-19.0392, -43.579) -> (-19.0617, -43.1585) projected
  line L488 (-19.0083, -44.0023) -> (-19.0392, -43.579) projected
  line L489 (-18.969, -44.4283) -> (-19.0083, -44.0023) projected
  line L490 (-18.9216, -44.8569) -> (-18.969, -44.4283) projected
  line L491 (-18.866, -45.2878) -> (-18.9216, -44.8569) projected
  line L492 (-18.8024, -45.721) -> (-18.866, -45.2878) projected
  line L493 (-18.7309, -46.1563) -> (-18.8024, -45.721) projected
  line L494 (-18.394, -46.2916) -> (-18.7309, -46.1563) projected
  line L495 (-18.0561, -46.4245) -> (-18.394, -46.2916) projected
  line L496 (-17.7172, -46.5548) -> (-18.0561, -46.4245) projected
  line L497 (-17.3775, -46.6827) -> (-17.7172, -46.5548) projected
  line L498 (-17.0368, -46.8081) -> (-17.3775, -46.6827) projected
  line L499 (-16.6952, -46.9311) -> (-17.0368, -46.8081) projected
  line L500 (-16.3527, -47.0515) -> (-16.6952, -46.9311) projected
  line L501 (-16.0093, -47.1694) -> (-16.3527, -47.0515) projected
  line L502 (-15.6651, -47.2849) -> (-16.0093, -47.1694) projected
  line L503 (-15.32, -47.3978) -> (-15.6651, -47.2849) projected
  line L504 (-14.9854, -47.1103) -> (-15.32, -47.3978) projected
  line L505 (-14.6582, -46.8193) -> (-14.9854, -47.1103) projected
  line L506 (-14.3387, -46.5249) -> (-14.6582, -46.8193) projected
  line L507 (-14.0269, -46.2271) -> (-14.3387, -46.5249) projected
  line L508 (-13.723, -45.926) -> (-14.0269, -46.2271) projected
  line L509 (-13.4272, -45.6216) -> (-13.723, -45.926) projected
  line L510 (-13.1396, -45.314) -> (-13.4272, -45.6216) projected
  line L511 (-12.8605, -45.0031) -> (-13.1396, -45.314) projected
  line L512 (-12.59, -44.689) -> (-12.8605, -45.0031) projected
  line L513 (-12.3286, -44.3718) -> (-12.59, -44.689) projected
  line L514 (-12.0764, -44.0514) -> (-12.3286, -44.3718) projected
  line L515 (-11.8338, -43.7278) -> (-12.0764, -44.0514) projected
  line L516 (-11.6012, -43.4011) -> (-11.8338, -43.7278) projected
  line L517 (-11.3792, -43.0711) -> (-11.6012, -43.4011) projected
  line L518 (-11.1684, -42.7378) -> (-11.3792, -43.0711) projected
  line L519 (-10.9697, -42.401) -> (-11.1684, -42.7378) projected
  line L520 (-10.7842, -42.0605) -> (-10.9697, -42.401) projected
  line L521 (-10.6138, -41.716) -> (-10.7842, -42.0605) projected
  line L522 (-10.4616, -41.3668) -> (-10.6138, -41.716) projected
  line L523 (-10.3363, -41.0107) -> (-10.4616, -41.3668) projected
  line L524 (-10.2574, -40.7427) -> (-10.3363, -41.0107) projected
  line L525 (-10.1693, -40.4859) -> (-10.2574, -40.7427) projected
  line L526 (-10.0741, -40.2401) -> (-10.1693, -40.4859) projected
  line L527 (-9.9747, -40.0046) -> (-10.0741, -40.2401) projected
  line L528 (-9.8655, -39.7811) -> (-9.9747, -40.0046) projected
  line L529 (-9.7467, -39.5697) -> (-9.8655, -39.7811) projected
  line L530 (-9.6179, -39.3708) -> (-9.7467, -39.5697) projected
  line L531 (-9.4853, -39.183) -> (-9.6179, -39.3708) projected
  line L532 (-9.3428, -39.0081) -> (-9.4853, -39.183) projected
  line L533 (-9.1886, -38.8469) -> (-9.3428, -39.0081) projected
  line L534 (-9.0298, -38.698) -> (-9.1886, -38.8469) projected
  line L535 (-8.8599, -38.5632) -> (-9.0298, -38.698) projected
  line L536 (-8.6799, -38.4428) -> (-8.8599, -38.5632) projected
  line L537 (-8.4928, -38.3367) -> (-8.6799, -38.4428) projected
  line L538 (-8.2917, -38.2471) -> (-8.4928, -38.3367) projected
  line L539 (-8.0839, -38.1732) -> (-8.2917, -38.2471) projected
  line L540 (-7.8581, -38.1187) -> (-8.0839, -38.1732) projected
  line L541 (-7.62, -38.0842) -> (-7.8581, -38.1187) projected
  line L542 (-7.347, -38.077) -> (-7.62, -38.0842) projected
  line L543 (-7.0016, -38.1122) -> (-7.347, -38.077) projected
  line L544 (-6.9471, -38.1222) -> (-7.0016, -38.1122) projected
  line L545 (-6.8925, -38.1321) -> (-6.9471, -38.1222) projected
  line L546 (-6.838, -38.1419) -> (-6.8925, -38.1321) projected
  line L547 (-6.7834, -38.1516) -> (-6.838, -38.1419) projected
  line L548 (-6.7289, -38.1613) -> (-6.7834, -38.1516) projected
  line L549 (-6.6743, -38.1709) -> (-6.7289, -38.1613) projected
  line L550 (-6.6197, -38.1804) -> (-6.6743, -38.1709) projected
  line L551 (-6.5651, -38.1898) -> (-6.6197, -38.1804) projected
  line L552 (-6.5105, -38.1992) -> (-6.5651, -38.1898) projected
  line L553 (-6.4558, -38.2084) -> (-6.5105, -38.1992) projected
  line L554 (-6.1191, -38.2935) -> (-6.4558, -38.2084) projected
  line L555 (-5.8651, -38.3936) -> (-6.1191, -38.2935) projected
  line L556 (-5.6532, -38.5075) -> (-5.8651, -38.3936) projected
  line L557 (-5.4597, -38.636) -> (-5.6532, -38.5075) projected
  line L558 (-5.2896, -38.7764) -> (-5.4597, -38.636) projected
  line L559 (-5.1313, -38.9295) -> (-5.2896, -38.7764) projected
  line L560 (-4.9918, -39.0931) -> (-5.1313, -38.9295) projected
  line L561 (-4.8638, -39.2678) -> (-4.9918, -39.0931) projected
  line L562 (-4.7503, -39.4526) -> (-4.8638, -39.2678) projected
  line L563 (-4.6519, -39.6468) -> (-4.7503, -39.4526) projected
  line L564 (-4.5622, -39.8511) -> (-4.6519, -39.6468) projected
  line L565 (-4.4881, -40.0641) -> (-4.5622, -39.8511) projected
  line L566 (-4.4278, -40.2859) -> (-4.4881, -40.0641) projected
  line L567 (-4.3747, -40.5169) -> (-4.4278, -40.2859) projected
  line L568 (-4.3353, -40.7562) -> (-4.3747, -40.5169) projected
  line L569 (-4.3093, -41.0036) -> (-4.3353, -40.7562) projected
  line L570 (-4.2964, -41.2588) -> (-4.3093, -41.0036) projected
  line L571 (-4.291, -41.5224) -> (-4.2964, -41.2588) projected
  line L572 (-4.2961, -41.7938) -> (-4.291, -41.5224) projected
  line L573 (-4.3135, -42.0727) -> (-4.2961, -41.7938) projected
  line L574 (-4.3176, -42.4502) -> (-4.3135, -42.0727) projected
  line L575 (-4.294, -42.8304) -> (-4.3176, -42.4502) projected
  line L576 (-4.2517, -43.2124) -> (-4.294, -42.8304) projected
  line L577 (-4.1939, -43.5958) -> (-4.2517, -43.2124) projected
  line L578 (-4.1223, -43.9802) -> (-4.1939, -43.5958) projected
  line L579 (-4.0382, -44.3655) -> (-4.1223, -43.9802) projected
  line L580 (-3.9425, -44.7515) -> (-4.0382, -44.3655) projected
  line L581 (-3.8357, -45.1381) -> (-3.9425, -44.7515) projected
  line L582 (-3.7184, -45.5251) -> (-3.8357, -45.1381) projected
  line L583 (-3.591, -45.9125) -> (-3.7184, -45.5251) projected
  line L584 (-3.4538, -46.3) -> (-3.591, -45.9125) projected
  line L585 (-3.3071, -46.6876) -> (-3.4538, -46.3) projected
  line L586 (-3.1511, -47.0752) -> (-3.3071, -46.6876) projected
  line L587 (-2.9861, -47.4626) -> (-3.1511, -47.0752) projected
  line L588 (-2.8122, -47.8499) -> (-2.9861, -47.4626) projected
  line L589 (-2.6297, -48.2368) -> (-2.8122, -47.8499) projected
  line L590 (-2.4385, -48.6232) -> (-2.6297, -48.2368) projected
  line L591 (-2.2389, -49.0092) -> (-2.4385, -48.6232) projected
  line L592 (-2.031, -49.3945) -> (-2.2389, -49.0092) projected
  line L593 (-1.8149, -49.7791) -> (-2.031, -49.3945) projected
  line L594 (-1.452, -49.791) -> (-1.8149, -49.7791) projected
  line L595 (-1.0891, -49.8003) -> (-1.452, -49.791) projected
  line L596 (-0.7261, -49.8069) -> (-1.0891, -49.8003) projected
  line L597 (-0.363, -49.8108) -> (-0.7261, -49.8069) projected
  line L598 (0, -49.8122) -> (-0.363, -49.8108) projected
  line L599 (0.363, -49.8108) -> (0, -49.8122) projected
  line L600 (0.7261, -49.8069) -> (0.363, -49.8108) projected
  line L601 (1.0891, -49.8003) -> (0.7261, -49.8069) projected
  line L602 (1.452, -49.791) -> (1.0891, -49.8003) projected
  line L603 (1.8149, -49.7791) -> (1.452, -49.791) projected
  line L604 (2.031, -49.3945) -> (1.8149, -49.7791) projected
  line L605 (2.2389, -49.0092) -> (2.031, -49.3945) projected
  line L606 (2.4385, -48.6232) -> (2.2389, -49.0092) projected
  line L607 (2.6297, -48.2368) -> (2.4385, -48.6232) projected
  line L608 (2.8122, -47.8499) -> (2.6297, -48.2368) projected
  line L609 (2.9861, -47.4626) -> (2.8122, -47.8499) projected
  line L610 (3.1511, -47.0752) -> (2.9861, -47.4626) projected
  line L611 (3.3071, -46.6876) -> (3.1511, -47.0752) projected
  line L612 (3.4538, -46.3) -> (3.3071, -46.6876) projected
  line L613 (3.591, -45.9125) -> (3.4538, -46.3) projected
  line L614 (3.7184, -45.5251) -> (3.591, -45.9125) projected
  line L615 (3.8357, -45.1381) -> (3.7184, -45.5251) projected
  line L616 (3.9425, -44.7515) -> (3.8357, -45.1381) projected
  line L617 (4.0382, -44.3655) -> (3.9425, -44.7515) projected
  line L618 (4.1223, -43.9802) -> (4.0382, -44.3655) projected
  line L619 (4.1939, -43.5958) -> (4.1223, -43.9802) projected
  line L620 (4.2517, -43.2124) -> (4.1939, -43.5958) projected
  line L621 (4.294, -42.8304) -> (4.2517, -43.2124) projected
  line L622 (4.3176, -42.4502) -> (4.294, -42.8304) projected
  line L623 (4.3135, -42.0727) -> (4.3176, -42.4502) projected
  line L624 (4.2961, -41.7938) -> (4.3135, -42.0727) projected
  line L625 (4.291, -41.5224) -> (4.2961, -41.7938) projected
  line L626 (4.2964, -41.2588) -> (4.291, -41.5224) projected
  line L627 (4.3093, -41.0036) -> (4.2964, -41.2588) projected
  line L628 (4.3353, -40.7562) -> (4.3093, -41.0036) projected
  line L629 (4.3747, -40.5169) -> (4.3353, -40.7562) projected
  line L630 (4.4278, -40.2859) -> (4.3747, -40.5169) projected
  line L631 (4.4881, -40.0641) -> (4.4278, -40.2859) projected
  line L632 (4.5622, -39.8511) -> (4.4881, -40.0641) projected
  line L633 (4.6519, -39.6468) -> (4.5622, -39.8511) projected
  line L634 (4.7503, -39.4526) -> (4.6519, -39.6468) projected
  line L635 (4.8638, -39.2678) -> (4.7503, -39.4526) projected
  line L636 (4.9918, -39.0931) -> (4.8638, -39.2678) projected
  line L637 (5.1313, -38.9295) -> (4.9918, -39.0931) projected
  line L638 (5.2896, -38.7764) -> (5.1313, -38.9295) projected
  line L639 (5.4597, -38.636) -> (5.2896, -38.7764) projected
  line L640 (5.6532, -38.5075) -> (5.4597, -38.636) projected
  line L641 (5.8651, -38.3936) -> (5.6532, -38.5075) projected
  line L642 (6.1191, -38.2935) -> (5.8651, -38.3936) projected
  line L643 (6.4558, -38.2084) -> (6.1191, -38.2935) projected
  line L644 (6.5105, -38.1992) -> (6.4558, -38.2084) projected
  line L645 (6.5651, -38.1898) -> (6.5105, -38.1992) projected
  line L646 (6.6197, -38.1804) -> (6.5651, -38.1898) projected
  line L647 (6.6743, -38.1709) -> (6.6197, -38.1804) projected
  line L648 (6.7289, -38.1613) -> (6.6743, -38.1709) projected
  line L649 (6.7834, -38.1516) -> (6.7289, -38.1613) projected
  line L650 (6.838, -38.1419) -> (6.7834, -38.1516) projected
  line L651 (6.8925, -38.1321) -> (6.838, -38.1419) projected
  line L652 (6.9471, -38.1222) -> (6.8925, -38.1321) projected
  line L653 (7.0016, -38.1122) -> (6.9471, -38.1222) projected
  line L654 (7.347, -38.077) -> (7.0016, -38.1122) projected
  line L655 (7.62, -38.0842) -> (7.347, -38.077) projected
  line L656 (7.8581, -38.1187) -> (7.62, -38.0842) projected
  line L657 (8.0839, -38.1732) -> (7.8581, -38.1187) projected
  line L658 (8.2917, -38.2471) -> (8.0839, -38.1732) projected
  line L659 (8.4928, -38.3367) -> (8.2917, -38.2471) projected
  line L660 (8.6799, -38.4428) -> (8.4928, -38.3367) projected
  line L661 (8.8599, -38.5632) -> (8.6799, -38.4428) projected
  line L662 (9.0298, -38.698) -> (8.8599, -38.5632) projected
  line L663 (9.1886, -38.8469) -> (9.0298, -38.698) projected
  line L664 (9.3428, -39.0081) -> (9.1886, -38.8469) projected
  line L665 (9.4853, -39.183) -> (9.3428, -39.0081) projected
  line L666 (9.6179, -39.3708) -> (9.4853, -39.183) projected
  line L667 (9.7467, -39.5697) -> (9.6179, -39.3708) projected
  line L668 (9.8655, -39.7811) -> (9.7467, -39.5697) projected
  line L669 (9.9747, -40.0046) -> (9.8655, -39.7811) projected
  line L670 (10.0741, -40.2401) -> (9.9747, -40.0046) projected
  line L671 (10.1693, -40.4859) -> (10.0741, -40.2401) projected
  line L672 (10.2574, -40.7427) -> (10.1693, -40.4859) projected
  line L673 (10.3363, -41.0107) -> (10.2574, -40.7427) projected
  line L674 (10.4616, -41.3668) -> (10.3363, -41.0107) projected
  line L675 (10.6138, -41.716) -> (10.4616, -41.3668) projected
  line L676 (10.7842, -42.0605) -> (10.6138, -41.716) projected
  line L677 (10.9697, -42.401) -> (10.7842, -42.0605) projected
  line L678 (11.1684, -42.7378) -> (10.9697, -42.401) projected
  line L679 (11.3792, -43.0711) -> (11.1684, -42.7378) projected
  line L680 (11.6012, -43.4011) -> (11.3792, -43.0711) projected
  line L681 (11.8338, -43.7278) -> (11.6012, -43.4011) projected
  line L682 (12.0764, -44.0514) -> (11.8338, -43.7278) projected
  line L683 (12.3286, -44.3718) -> (12.0764, -44.0514) projected
  line L684 (12.59, -44.689) -> (12.3286, -44.3718) projected
  line L685 (12.8605, -45.0031) -> (12.59, -44.689) projected
  line L686 (13.1396, -45.314) -> (12.8605, -45.0031) projected
  line L687 (13.4272, -45.6216) -> (13.1396, -45.314) projected
  line L688 (13.723, -45.926) -> (13.4272, -45.6216) projected
  line L689 (14.0269, -46.2271) -> (13.723, -45.926) projected
  line L690 (14.3387, -46.5249) -> (14.0269, -46.2271) projected
  line L691 (14.6582, -46.8193) -> (14.3387, -46.5249) projected
  line L692 (14.9854, -47.1103) -> (14.6582, -46.8193) projected
  line L693 (15.32, -47.3978) -> (14.9854, -47.1103) projected
  line L694 (15.6651, -47.2849) -> (15.32, -47.3978) projected
  line L695 (16.0093, -47.1694) -> (15.6651, -47.2849) projected
  line L696 (16.3527, -47.0515) -> (16.0093, -47.1694) projected
  line L697 (16.6952, -46.9311) -> (16.3527, -47.0515) projected
  line L698 (17.0368, -46.8081) -> (16.6952, -46.9311) projected
  line L699 (17.3775, -46.6827) -> (17.0368, -46.8081) projected
  line L700 (17.7172, -46.5548) -> (17.3775, -46.6827) projected
  line L701 (18.0561, -46.4245) -> (17.7172, -46.5548) projected
  line L702 (18.394, -46.2916) -> (18.0561, -46.4245) projected
  line L703 (18.7309, -46.1563) -> (18.394, -46.2916) projected
  line L704 (18.8024, -45.721) -> (18.7309, -46.1563) projected
  line L705 (18.866, -45.2878) -> (18.8024, -45.721) projected
  line L706 (18.9216, -44.8569) -> (18.866, -45.2878) projected
  line L707 (18.969, -44.4283) -> (18.9216, -44.8569) projected
  line L708 (19.0083, -44.0023) -> (18.969, -44.4283) projected
  line L709 (19.0392, -43.579) -> (19.0083, -44.0023) projected
  line L710 (19.0617, -43.1585) -> (19.0392, -43.579) projected
  line L711 (19.0757, -42.7409) -> (19.0617, -43.1585) projected
  line L712 (19.081, -42.3265) -> (19.0757, -42.7409) projected
  line L713 (19.0774, -41.9154) -> (19.081, -42.3265) projected
  line L714 (19.0647, -41.5079) -> (19.0774, -41.9154) projected
  line L715 (19.0425, -41.1041) -> (19.0647, -41.5079) projected
  line L716 (19.0107, -40.7043) -> (19.0425, -41.1041) projected
  line L717 (18.9686, -40.3088) -> (19.0107, -40.7043) projected
  line L718 (18.9158, -39.9179) -> (18.9686, -40.3088) projected
  line L719 (18.8516, -39.5322) -> (18.9158, -39.9179) projected
  line L720 (18.7748, -39.1522) -> (18.8516, -39.5322) projected
  line L721 (18.6839, -38.7788) -> (18.7748, -39.1522) projected
  line L722 (18.576, -38.4134) -> (18.6839, -38.7788) projected
  line L723 (18.4431, -38.0601) -> (18.576, -38.4134) projected
  line L724 (18.3313, -37.804) -> (18.4431, -38.0601) projected
  line L725 (18.2337, -37.5507) -> (18.3313, -37.804) projected
  line L726 (18.1486, -37.3012) -> (18.2337, -37.5507) projected
  line L727 (18.0734, -37.0569) -> (18.1486, -37.3012) projected
  line L728 (18.0133, -36.8155) -> (18.0734, -37.0569) projected
  line L729 (17.9685, -36.5772) -> (18.0133, -36.8155) projected
  line L730 (17.9393, -36.342) -> (17.9685, -36.5772) projected
  line L731 (17.9202, -36.1129) -> (17.9393, -36.342) projected
  line L732 (17.9169, -35.8874) -> (17.9202, -36.1129) projected
  line L733 (17.9314, -35.6648) -> (17.9169, -35.8874) projected
  line L734 (17.9574, -35.4486) -> (17.9314, -35.6648) projected
  line L735 (18.0008, -35.2362) -> (17.9574, -35.4486) projected
  line L736 (18.0614, -35.0282) -> (18.0008, -35.2362) projected
  line L737 (18.1365, -34.8267) -> (18.0614, -35.0282) projected
  line L738 (18.2329, -34.6288) -> (18.1365, -34.8267) projected
  line L739 (18.3447, -34.4386) -> (18.2329, -34.6288) projected
  line L740 (18.4826, -34.2517) -> (18.3447, -34.4386) projected
  line L741 (18.6427, -34.0722) -> (18.4826, -34.2517) projected
  line L742 (18.8473, -33.8913) -> (18.6427, -34.0722) projected
  line L743 (19.1345, -33.6962) -> (18.8473, -33.8913) projected
  line L744 (19.1827, -33.6688) -> (19.1345, -33.6962) projected
  line L745 (19.2308, -33.6413) -> (19.1827, -33.6688) projected
  line L746 (19.2789, -33.6138) -> (19.2308, -33.6413) projected
  line L747 (19.327, -33.5862) -> (19.2789, -33.6138) projected
  line L748 (19.375, -33.5585) -> (19.327, -33.5862) projected
  line L749 (19.423, -33.5307) -> (19.375, -33.5585) projected
  line L750 (19.4709, -33.5029) -> (19.423, -33.5307) projected
  line L751 (19.5188, -33.475) -> (19.4709, -33.5029) projected
  line L752 (19.5667, -33.4471) -> (19.5188, -33.475) projected
  line L753 (19.6145, -33.4191) -> (19.5667, -33.4471) projected
  line L754 (19.9271, -33.2679) -> (19.6145, -33.4191) projected
  line L755 (20.186, -33.1812) -> (19.9271, -33.2679) projected
  line L756 (20.4215, -33.1323) -> (20.186, -33.1812) projected
  line L757 (20.6524, -33.1063) -> (20.4215, -33.1323) projected
  line L758 (20.8729, -33.1046) -> (20.6524, -33.1063) projected
  line L759 (21.0926, -33.12) -> (20.8729, -33.1046) projected
  line L760 (21.3046, -33.1558) -> (21.0926, -33.12) projected
  line L761 (21.515, -33.2073) -> (21.3046, -33.1558) projected
  line L762 (21.7207, -33.2758) -> (21.515, -33.2073) projected
  line L763 (21.9209, -33.3615) -> (21.7207, -33.2758) projected
  line L764 (22.121, -33.4602) -> (21.9209, -33.3615) projected
  line L765 (22.3146, -33.5758) -> (22.121, -33.4602) projected
  line L766 (22.5034, -33.7069) -> (22.3146, -33.5758) projected
  line L767 (22.6925, -33.8498) -> (22.5034, -33.7069) projected
  line L768 (22.8765, -34.0078) -> (22.6925, -33.8498) projected
  line L769 (23.0555, -34.1805) -> (22.8765, -34.0078) projected
  line L770 (23.2294, -34.3678) -> (23.0555, -34.1805) projected
  line L771 (23.403, -34.5662) -> (23.2294, -34.3678) projected
  line L772 (23.5736, -34.7774) -> (23.403, -34.5662) projected
  line L773 (23.7394, -35.0022) -> (23.5736, -34.7774) projected
  line L774 (23.979, -35.294) -> (23.7394, -35.0022) projected
  line L775 (24.2415, -35.5701) -> (23.979, -35.294) projected
  line L776 (24.5194, -35.8356) -> (24.2415, -35.5701) projected
  line L777 (24.8101, -36.092) -> (24.5194, -35.8356) projected
  line L778 (25.1121, -36.3405) -> (24.8101, -36.092) projected
  line L779 (25.4241, -36.5817) -> (25.1121, -36.3405) projected
  line L780 (25.7456, -36.8158) -> (25.4241, -36.5817) projected
  line L781 (26.0759, -37.0434) -> (25.7456, -36.8158) projected
  line L782 (26.4145, -37.2644) -> (26.0759, -37.0434) projected
  line L783 (26.7611, -37.4792) -> (26.4145, -37.2644) projected
  line L784 (27.1153, -37.6879) -> (26.7611, -37.4792) projected
  line L785 (27.4768, -37.8905) -> (27.1153, -37.6879) projected
  line L786 (27.8455, -38.0872) -> (27.4768, -37.8905) projected
  line L787 (28.2209, -38.2779) -> (27.8455, -38.0872) projected
  line L788 (28.603, -38.4628) -> (28.2209, -38.2779) projected
  line L789 (28.9916, -38.6418) -> (28.603, -38.4628) projected
  line L790 (29.3864, -38.815) -> (28.9916, -38.6418) projected
  line L791 (29.7874, -38.9823) -> (29.3864, -38.815) projected
  line L792 (30.1943, -39.1439) -> (29.7874, -38.9823) projected
  line L793 (30.6071, -39.2996) -> (30.1943, -39.1439) projected
  line L794 (30.8927, -39.0755) -> (30.6071, -39.2996) projected
  line L795 (31.1767, -38.8493) -> (30.8927, -39.0755) projected
  line L796 (31.459, -38.621) -> (31.1767, -38.8493) projected
  line L797 (31.7397, -38.3907) -> (31.459, -38.621) projected
  line L798 (32.0186, -38.1583) -> (31.7397, -38.3907) projected
  line L799 (32.2959, -37.924) -> (32.0186, -38.1583) projected
  line L800 (32.5715, -37.6876) -> (32.2959, -37.924) projected
  line L801 (32.8453, -37.4492) -> (32.5715, -37.6876) projected
  line L802 (33.1173, -37.2088) -> (32.8453, -37.4492) projected
  line L803 (33.3877, -36.9664) -> (33.1173, -37.2088) projected
  line L804 (33.306, -36.5329) -> (33.3877, -36.9664) projected
  line L805 (33.2176, -36.1041) -> (33.306, -36.5329) projected
  line L806 (33.1224, -35.6801) -> (33.2176, -36.1041) projected
  line L807 (33.0204, -35.2612) -> (33.1224, -35.6801) projected
  line L808 (32.9116, -34.8475) -> (33.0204, -35.2612) projected
  line L809 (32.7959, -34.4391) -> (32.9116, -34.8475) projected
  line L810 (32.6732, -34.0362) -> (32.7959, -34.4391) projected
  line L811 (32.5436, -33.639) -> (32.6732, -34.0362) projected
  line L812 (32.4068, -33.2478) -> (32.5436, -33.639) projected
  line L813 (32.2628, -32.8628) -> (32.4068, -33.2478) projected
  line L814 (32.1115, -32.4841) -> (32.2628, -32.8628) projected
  line L815 (31.9525, -32.1123) -> (32.1115, -32.4841) projected
  line L816 (31.7858, -31.7475) -> (31.9525, -32.1123) projected
  line L817 (31.6111, -31.3902) -> (31.7858, -31.7475) projected
  line L818 (31.4278, -31.041) -> (31.6111, -31.3902) projected
  line L819 (31.2355, -30.7005) -> (31.4278, -31.041) projected
  line L820 (31.0334, -30.3697) -> (31.2355, -30.7005) projected
  line L821 (30.8202, -30.0499) -> (31.0334, -30.3697) projected
  line L822 (30.5939, -29.7434) -> (30.8202, -30.0499) projected
  line L823 (30.3482, -29.4569) -> (30.5939, -29.7434) projected
  line L824 (30.1555, -29.2545) -> (30.3482, -29.4569) projected
  line L825 (29.9772, -29.0498) -> (30.1555, -29.2545) projected
  line L826 (29.8119, -28.8444) -> (29.9772, -29.0498) projected
  line L827 (29.6577, -28.6406) -> (29.8119, -28.8444) projected
  line L828 (29.5186, -28.4343) -> (29.6577, -28.6406) projected
  line L829 (29.395, -28.2257) -> (29.5186, -28.4343) projected
  line L830 (29.2872, -28.0147) -> (29.395, -28.2257) projected
  line L831 (29.1908, -27.806) -> (29.2872, -28.0147) projected
  line L832 (29.1106, -27.5952) -> (29.1908, -27.806) projected
  line L833 (29.0481, -27.381) -> (29.1106, -27.5952) projected
  line L834 (28.9985, -27.169) -> (29.0481, -27.381) projected
  line L835 (28.9667, -26.9545) -> (28.9985, -27.169) projected
  line L836 (28.9525, -26.7384) -> (28.9667, -26.9545) projected
  line L837 (28.9541, -26.5234) -> (28.9525, -26.7384) projected
  line L838 (28.9771, -26.3044) -> (28.9541, -26.5234) projected
  line L839 (29.0171, -26.0875) -> (28.9771, -26.3044) projected